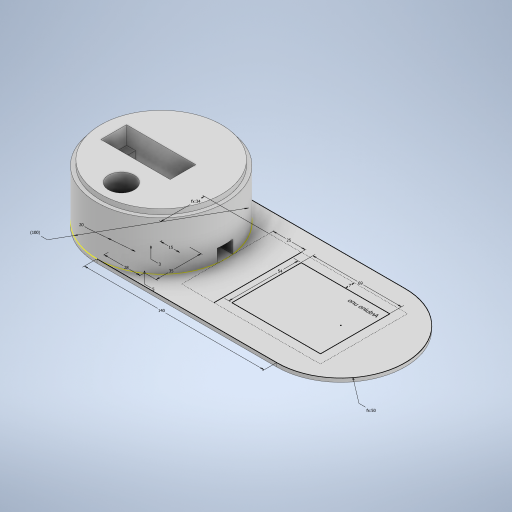
# Autodesk Inventor part: Base v0,1
Saved by Autodesk Inventor 2023 (Build 270158000, 158)
## iProperties
Created: 2024-06-24
Part Number: Base v0,1
Material: Generic
Document SubType Name: Modeling
Designer: Swoby
Density: 1 g/cm^3
Appearance: Default
Author: Swoby
Autodesk Inventor part; units mm, degrees
ref_plane "YZ Plane" through (0, 0, 0) normal (1, 0, 0) x (0, 1, 0)
ref_plane "XZ Plane" through (0, 0, 0) normal (0, 1, 0) x (-1, 0, 0)
ref_plane "XY Plane" through (0, 0, 0) normal (0, 0, 1) x (1, 0, 0)
sketch "Sketch1" plane through (0, 0, 0) normal (0, 0, 1) x (1, 0, 0)
  line L0 (0, 0) -> (50, 0)
  line L1 (50, 0) -> (50, 38)
  line L2 (50, 38) -> (0, 38)
  line L3 (0, 38) -> (0, 0)
  dimension "d0" = 100
  dimension "d1" = 38
  constraints: 8 end point, 2 parallel, 1 horizontal, 1 perpendicular
  measures "d0" diameter of L1 L3
  measures "d1" distance of L0.end L1.end
revolve "Revolution1" add sketch "Sketch1" angle 360 about axis through (0, 38, 0) along (0, -1, 0)
sketch "Sketch2" plane through (0, 38, 0) normal (0, 1, 0) x (1, 0, 0)
  line L0 (-30, 10) -> (10, 10)
  line L1 (10, 10) -> (10, -10)
  line L2 (10, -10) -> (-30, -10)
  line L3 (-30, -10) -> (-30, 10)
  line L4 (10, -10) -> (17, -10)
  line L5 (17, -10) -> (17, 10)
  line L6 (17, 10) -> (10, 10)
  line L7 (10, 10) -> (10, -10)
  line L8 (-30, -10) -> (-37, -10)
  line L9 (-37, -10) -> (-37, 10)
  line L10 (-37, 10) -> (-30, 10)
  line L11 (-30, 10) -> (-30, -10)
  point P0 (0, 0)
  dimension "d3" = 10
  dimension "d4" = 40
  dimension "d5" = 20
  dimension "d6" = 10
  dimension "d7" = 7
  dimension "d8" = 7
  constraints: 24 end point, 6 parallel, 3 horizontal, 3 perpendicular, 2 point on line
  measures "d3" distance from line of point (0, 0) L1
  measures "d4" distance of L0.start L0.end
  measures "d5" distance of L0.end L1.end
  measures "d6" distance from line of L0 point (0, 0)
  measures "d7" distance of L6.end L5.end
  measures "d8" distance of L9.end L10.end
extrude "Extrusion1" cut sketch "Sketch2" against normal blind 38 contours L0 L1 L2 L3
extrude "Extrusion2" cut sketch "Sketch2" against normal blind 10 contours L3 L8 L9 L10 | L6 L5 L4 L1
sketch "Sketch3" plane through (0, 0, 0) normal (0, -1, 0) x (1, 0, 0)
  line L0 (10, 10) -> (10, -10) projected
  line L1 (10, 6) -> (10, -6)
  line L2 (10, -6) -> (49.6387, -6)
  line L3 (10, 6) -> (49.6387, 6)
  circle A0 centre (0, 0) radius 50 projected
  point P0 (0, 0)
  dimension "d13" = 12
  dimension "d14" = 6
  constraints: 6 end point, 2 point on circle, 2 point on line, 1 horizontal, 1 parallel
  measures "d13" distance between parallel lines of L2 L3
  measures "d14" distance from line of point (0, 0) L3
extrude "Extrusion3" cut sketch "Sketch3" against normal blind 10 contours L3 A0 L2 L0 picked at (23.3333, 0)
sketch "Sketch4" plane through (-30, 0, -10) normal (0, -1, 0) x (1, 0, 0)
  line L0 (181, -17) -> (112, -17)
  line L1 (112, -17) -> (112, 37)
  line L2 (112, 37) -> (181, 37)
  line L3 (181, 37) -> (181, -17)
  line L4 (181, -17) -> (112, -17) construction
  line L5 (112, -17) -> (112, 37) construction
  line L6 (112, 37) -> (181, 37) construction
  line L7 (181, 37) -> (181, -17) construction
  line L8 (105, -24) -> (188, -24) construction
  line L9 (188, -24) -> (188, 44) construction
  line L10 (188, 44) -> (105, 44) construction
  line L11 (105, 44) -> (105, -24) construction
  line L12 (105, 44) -> (80, 44) construction
  line L13 (80, 44) -> (80, -24) construction
  line L14 (80, -24) -> (105, -24) construction
  line L15 (105, -24) -> (105, 44)
  arc A0 (79.6387, 4) -> (79.6387, 16) centre (30, 10) ccw projected
  arc A1 (79.6387, 16) -> (79.6387, 4) centre (30, 10) ccw projected
  circle A2 centre (30, 41) radius 10
  line L16 (30, 51) -> (53, 51)
  line L17 (58, 46) -> (58, 16)
  line L18 (40, 16) -> (79.6387, 16) projected
  line L19 (43, 28) -> (43, 16)
  line L20 (30, 10) -> (30, 41) construction
  arc A3 (58, 46) -> (53, 51) centre (53, 46) ccw
  arc A4 (43, 28) -> (40, 31) centre (40, 28) ccw
  circle A5 centre (30, 10) radius 50 projected
  line L21 (30, 60) -> (170, 60)
  line L22 (30, -40) -> (170, -40)
  arc A6 (170, -40) -> (170, 60) centre (170, 10) ccw
  line L23 (40, 31) -> (30, 31)
  point P0 (58, 51)
  dimension "d17" = 69
  dimension "d18" = 54
  dimension "d19" = 7
  dimension "d20" = 25
  dimension "d21" = 34
  dimension "d22" = 20
  dimension "d23" = 15
  dimension "d25" = 28
  dimension "d26" = 35
  dimension "d27" = 5
  dimension "d28" = 3
  dimension "d33" = 100
  dimension "d34" = 50
  dimension "d35" = 140
  constraints: 38 end point, 10 point on circle, 10 tangent, 9 point on line, 7 parallel, 5 horizontal, 5 perpendicular, 4 centre point, 1 coincident, 1 vertical, 5 other
  measures "d17" distance of L0.start L0.end
  measures "d18" distance of L0.end L1.end
  measures "d19" distance between parallel lines of L0 L8
  measures "d20" distance of L13.end L14.end
  measures "d21" distance from line of L14 point (30, 10)
  measures "d22" diameter of A2
  measures "d23" distance between parallel lines of L17 L19
  measures "d25" distance of L16.start point (58, 51)
  measures "d26" distance of point (58, 51) L17.end
  measures "d27" radius of A3
  measures "d28" radius of A4
  measures "d33" diameter of A5
  measures "d34" radius of A6
  measures "d35" distance of L21.start L21.end
extrude "Extrusion4" cut sketch "Sketch4" against normal up to surface (10 mm away) contours A2 | A2 L16 A3 L17 L18 L19 A4 L23
sketch "Sketch5" plane through (0, 10, 0) normal (0, -1, 0) x (1, 0, 0)
  circle A0 centre (0, 31) radius 10
  arc A1 (0, 41) -> (0, 21) centre (0, 31) ccw projected
  point P0 (0, 0)
  dimension "d39" = 20
  constraints: 1 centre point, 1 coincident
  measures "d39" diameter of A0
extrude "Extrusion5" cut sketch "Sketch5" against normal through all
extrude "Extrusion6" add sketch "Sketch4" along normal blind 3 contours L0 L1 L2 L3 | A1 A0 | A0 A1 L21 A6 L22 | A2 | A2 L16 A3 L17 L18 L19 A4 L23
sketch "Sketch6" plane through (0, 38, 0) normal (0, 1, 0) x (1, 0, 0)
  line L0 (-37, -10) -> (-37, 10) projected
  line L1 (17, -10) -> (-37, -10) projected
  line L2 (-37, 10) -> (17, 10) projected
  line L3 (17, 10) -> (17, -10) projected
  circle A0 centre (0, -31) radius 10 projected
  circle A1 centre (0, -31) radius 10 projected
  line L4 (17, -10) -> (-37, -10) projected
  line L5 (-37, -10) -> (-37, 10) projected
  line L6 (-37, 10) -> (17, 10) projected
  line L7 (17, 10) -> (17, -10) projected
  circle A2 centre (0, 0) radius 50 projected
  circle A3 centre (0, 0) radius 47
  point P0 (0, 0)
  dimension "d40" = 94
  constraints: 1 centre point, 1 coincident
  measures "d40" diameter of A3
extrude "Extrusion7" add sketch "Sketch6" along normal blind 4 contours A3
equation "\"d14\" = 0.5 * d13"
equation "\"d21\" = d19 + 0.5 * d18"
equation "\"d34\" = 0.5 * d33"
equation "\"d39\" = d22"
body "Solid1"
